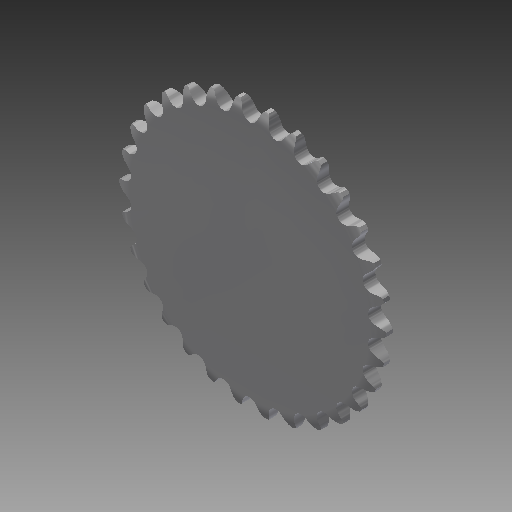
# Autodesk Inventor part: Sprocket1
Saved by Autodesk Inventor 2019 (Build 230136000, 136)
## iProperties
Created: 2019-11-15
Part Number: Sprocket1
Material: Steel
Document SubType Name: Modeling
Designer: Domenico
Density: 1 g/cm^3
Appearance: Steel
CustomPartVersion: 1
Author: Domenico
Autodesk Inventor part; units mm, degrees
ref_plane "YZ Plane" through (0, 0, 0) normal (1, 0, 0) x (0, 1, 0)
ref_plane "XZ Plane" through (0, 0, 0) normal (0, 1, 0) x (-1, 0, 0)
sketch "Theoretical Tooth Profile" plane through (0, 0, 0) normal (0, 0, 1) x (1, 0, 0)
  circle A0 centre (0, 0) radius 45.5618 construction
  line L0 (0, 0) -> (0, 45.5618) construction
  line L1 (0, 0) -> (9.4728, 44.5661) construction
  circle A1 centre (0, 0) radius 48.1697
  arc A2 (-2.0691, 44.0026) -> (2.0691, 44.0026) centre (0, 45.5618) ccw
  line L2 (0, 45.5618) -> (9.4728, 44.5661) construction
  line L3 (0, 45.5618) -> (3.2457, 48.0075) construction
  line L4 (3.2457, 48.0075) -> (-2.9727, 45.6371) construction
  arc A3 (4.4114, 47.9672) -> (3.2204, 46.287) centre (7.073, 44.8183) ccw
  arc A4 (-3.2204, 46.287) -> (-4.4114, 47.9672) centre (-7.073, 44.8183) ccw
  line L5 (-7.073, 44.8183) -> (-3.2204, 46.287) construction
  arc A5 (-2.9727, 45.6371) -> (-2.0691, 44.0026) centre (3.2457, 48.0075) ccw
  line L6 (-2.9727, 45.6371) -> (-3.2204, 46.287)
  arc A6 (2.0691, 44.0026) -> (2.9727, 45.6371) centre (-3.2457, 48.0075) ccw
  line L7 (3.2204, 46.287) -> (2.9727, 45.6371)
  line L8 (0, 0) -> (5.0351, 47.9058) construction
  point P0 (4.7364, 45.0639)
  dimension "d0" = 91.1235
  dimension "d2" = 12
  dimension "d3" = 2.5908
  dimension "d10" = 127
  dimension "d11" = 16.133
  dimension "d12" = 4.064
  dimension "d13" = 6.6548
  dimension "d14" = 7.112
  dimension "d23" = 2.8575
  constraints: 18 end point, 15 point on circle, 7 centre point, 3 coincident, 3 point on line, 3 symmetric about line, 3 tangent, 1 equal radius, 1 midpoint, 1 parallel, 1 vertical, 1 other
  measures "d0" diameter of A0
  measures "d2" angle of L1 L0
  measures "d3" radius of A2
  measures "d10" angle of L3 L0
  measures "d11" angle of L4 L3
  measures "d12" distance of L2.start L3.end
  measures "d13" distance of L3.end L4.end
  measures "d14" distance of A3.centre L0.end
  measures "d23" distance from line of L8.end L2
sketch "Tooth Profile" plane through (0, 0, 0) normal (0, 0, 1) x (1, 0, 0)
  arc A0 (-2.4105, 44.6122) -> (2.4105, 44.6122) centre (0, 45.5618) ccw
  arc A1 (4.1385, 47.9915) -> (2.4105, 44.6122) centre (20.5604, 37.4628) ccw
  arc A2 (-2.4105, 44.6122) -> (-4.1385, 47.9915) centre (-20.5604, 37.4628) ccw
  line L0 (0, 0) -> (0, 45.5618) construction
  line L1 (0, 45.5618) -> (2.4105, 44.6122) construction
  line L2 (0, 45.5618) -> (-2.4105, 44.6122) construction
  circle A3 centre (0, 0) radius 48.1697 projected
  dimension "d44" = 137
  dimension "d45" = 19.5072
  dimension "d46" = 2.5908
  constraints: 9 point on circle, 6 end point, 3 centre point, 2 tangent, 1 coincident, 1 equal radius, 1 vertical, 1 other
  measures "d44" angle of L2 L1
  measures "d45" radius of A1
  measures "d46" radius of A0
sketch "Section Profile" plane through (0, 0, 0) normal (1, 0, 0) x (0, 1, 0)
  line L0 (48.1697, 0) -> (-48.1697, 0) projected
  line L1 (39.7877, 2.2967) -> (-39.7877, 2.2967)
  line L2 (-39.7877, 2.2967) -> (-39.7877, -2.2967)
  line L3 (-39.7877, -2.2967) -> (39.7877, -2.2967)
  line L4 (39.7877, -2.2967) -> (39.7877, 2.2967)
  line L5 (39.7877, 2.2967) -> (48.1697, 2.2967) construction
  line L6 (48.1697, 2.2967) -> (48.1697, -2.2967) construction
  line L7 (48.1697, -2.2967) -> (39.7877, -2.2967) construction
  line L8 (39.7877, -2.2967) -> (39.7877, 2.2967)
  arc A0 (48.1697, 1.106) -> (43.406, 2.2967) centre (43.406, -7.8284) ccw
  arc A1 (43.406, -2.2967) -> (48.1697, -1.106) centre (43.406, 7.8284) ccw
  line L9 (43.406, 2.2967) -> (0, 2.2967)
  line L10 (0, 2.2967) -> (0, -2.2967)
  line L11 (0, -2.2967) -> (43.406, -2.2967)
  line L12 (0, 2.2967) -> (0, -2.2967)
  line L13 (48.1697, 1.106) -> (48.1697, -1.106)
  point P0 (0, 0)
  point P1 (0, 0)
  dimension "d30" = 4.5933
  dimension "d31" = 79.5753
  dimension "d32" = 4.5933
  dimension "d33" = 1.1906
  dimension "d34" = 10.1251
  dimension "d43" = 2.2967
  constraints: 26 end point, 7 midpoint, 5 perpendicular, 4 parallel, 4 point on circle, 3 point on line, 3 symmetric about line, 2 centre point, 2 horizontal, 2 tangent, 1 collinear, 1 other
  measures "d30" distance between parallel lines of L7 L5
  measures "d31" distance between parallel lines of L2 L4
  measures "d32" distance between parallel lines of L3 L1
  measures "d33" distance from line of L13.start L5
  measures "d34" radius of A0
  measures "d43" distance between parallel lines of L3 L0
revolve "Shroud" add sketch "Section Profile" angle 360 about axis through (0, 0, 2.2967) along (0, 0, -1) contours L10 L3 L2 L0 | L0 L2 L1 L10
revolve "Strand" add sketch "Section Profile" angle 360 about axis through (0, 0, 2.2967) along (0, 0, -1) contours L13 A1 L11 L4 L0 | L0 L4 L9 A0 L13 | L4 L3 L10 L0 | L0 L10 L1 L4
pattern_of_one "Strand Pattern"
extrude "Theoretical Tooth" cut sketch "Theoretical Tooth Profile" along normal through all both and the other way through all contours A3 L7 A6 A2 A5 L6 A4 A1 picked at (-0.4908, 45.7279)
extrude "Tooth" [suppressed]
pattern_circular "Tooth Pattern" count 30 over 360 about axis through (0, 0, -10) along (0, 0, 1) of "Theoretical Tooth"
ref_plane "Timing Plane" through (0, 45.5618, 0) normal (1, 0, 0) x (0, 1, 0)
equation "\"d3\" = 0.5 * da_Dr + da_SC"
equation "\"d12\" = 0.8 * da_Dr"
equation "\"d13\" = 1.3 * da_Dr + da_SC"
equation "\"d14\" = 1.4 * da_Dr"
equation "\"d23\" = da_Ha"
equation "\"d44\" = da_Alfa"
equation "\"d45\" = da_Re"
equation "\"d46\" = da_Ri"
equation "\"d30\" = da_Bf"
equation "\"d31\" = da_Ds"
equation "\"d32\" = da_Bs"
equation "\"d33\" = da_Ba"
equation "\"d34\" = da_Rx"
equation "\"d40\" = da_pt"
equation "\"form_type\" = 0"
equation "\"da_p\" = 9.525"
equation "\"da_Dr\" = 5.08"
equation "\"da_SC\" = 0.0508"
equation "\"da_Ha\" = 2.8575"
equation "\"da_pt\" = 10.1346"
equation "\"da_Bf\" = 4.59334"
equation "\"da_Ba\" = 1.19063"
equation "\"da_Rx\" = 10.12508"
equation "\"da_Ra\" = 0.381"
equation "\"da_Bs\" = 4.59334"
equation "\"da_Ds\" = 79.57532"
equation "\"da_Re\" = 19.5072"
equation "\"da_Ri\" = 2.5908"
equation "\"da_Alfa\" = 137deg"
body "Solid1"
